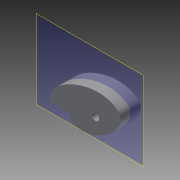
# Autodesk Inventor part: cam 3
Saved by Autodesk Inventor 2014 (Build 180170000, 170)
## iProperties
Created: 2014-05-19
Part Number: cam 3
Material: Generic
Document SubType Name: Modeling
Designer: jyesowitz
Density: 1 g/cm^3
Appearance: Default
Author: jyesowitz
Autodesk Inventor part; units mm, degrees
ref_plane "YZ Plane" through (0, 0, 0) normal (1, 0, 0) x (0, 1, 0)
ref_plane "XZ Plane" through (0, 0, 0) normal (0, 1, 0) x (-1, 0, 0)
ref_plane "XY Plane" through (0, 0, 0) normal (0, 0, 1) x (1, 0, 0)
sketch "Sketch1" plane through (0, 0, 0) normal (0, 0, 1) x (1, 0, 0)
  ellipse E0 centre (0, 0) end of major axis (30.3302, 18.3679) minor radius 18.4658 (-31.8027, -12.8271) -> (27.6607, 21.2638) ccw
  line L0 (27.6607, 21.2638) -> (-2.6708, 43.6957) construction
  line L1 (-2.6708, 43.6957) -> (-60.1955, 10.9449) construction
  line L2 (-60.1955, 10.9449) -> (-61.1401, -3.4433) construction
  line L3 (-61.1401, -3.4433) -> (-55.4573, -12.8271) construction
  spline S0 degree 4 poles (27.6607, 21.2638) (-2.6708, 43.6957) (-60.1955, 10.9449) (-61.1401, -3.4433) (-55.4573, -12.8271) knots 1 1 1 1 1 2 2 2 2 2
  line L4 (-55.4573, -12.8271) -> (-31.8027, -12.8271)
  circle A0 centre (0, 0) radius 4.7625
  point P0 (-43.63, -12.8271)
  dimension "d7" = 35.4584
  dimension "d13" = 18.4658
  dimension "d0" = 56.9214
  dimension "d2" = 37.7252
  dimension "d3" = 66.1944
  dimension "d4" = 14.4192
  dimension "d5" = 10.9704
  dimension "d6" = 34.2921
  dimension "d9" = 113.861
  dimension "d10" = 43.6957
  dimension "d14" = 9.525
  constraints: 2 coincident, 2 end point, 1 centre point, 1 horizontal, 1 midpoint, 9 other
  measures "d0" distance of L3.end point (0, 0)
  measures "d2" distance of L0.start L0.end
  measures "d3" distance of L0.end L1.end
  measures "d4" distance of L1.end L2.end
  measures "d5" distance of L2.end L3.end
  measures "d6" distance of point (0, 0) L4.end
  measures "d9" angle of L1 L0
  measures "d10" vertical distance of point (0, 0) L0.end
  measures "d14" diameter of A0
extrude "Extrusion1" add sketch "Sketch1" against normal blind 25.4
ref_plane "Work Plane1" through (0, 0, -12.7) normal (0, 0, -1) x (-1, 0, 0)
body "Solid1"
